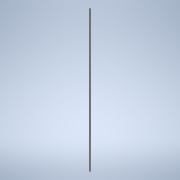
# Autodesk Inventor part: ball screw
Saved by Autodesk Inventor 2020 (Build 240168000, 168)
## iProperties
Created: 2020-07-28
Part Number: ball screw
Material: Stainless Steel
Document SubType Name: Modeling
Designer: Vikki
Density: 8 g/cm^3
Appearance: Semi-Polished
Mass: 1603.28 g
Surface Area: 506.216 cm^2
Volume: 200.409 cm^3
Author: Vikki
Autodesk Inventor part; units mm, degrees
ref_plane "YZ Plane" through (0, 0, 0) normal (1, 0, 0) x (0, 1, 0)
ref_plane "XZ Plane" through (0, 0, 0) normal (0, 1, 0) x (-1, 0, 0)
ref_plane "XY Plane" through (0, 0, 0) normal (0, 0, 1) x (1, 0, 0)
sketch "Sketch1" plane through (0, 0, 0) normal (0, 1, 0) x (-1, 0, 0)
  circle A0 centre (0, 0) radius 5
  dimension "d0" = 10
  constraints: 1 centre point, 1 coincident
  measures "d0" diameter of A0
extrude "Extrusion1" add sketch "Sketch1" along normal blind 1000
sketch "Sketch2" plane through (0, 1000, 0) normal (0, 1, 0) x (1, 0, 0)
  circle A0 centre (0, 0) radius 5 projected
  circle A1 centre (0, 0) radius 5 projected
  line L0 (5, 0) -> (5, 0)
  line L1 (0, 0) -> (0, 5)
  point P0 (5, 6.245)
  point P1 (5, -6.245)
  dimension "d3" = 5
  constraints: 4 end point, 2 point on circle, 1 parallel, 1 vertical
  measures "d3" distance from line of L0 point (0, 0)
extrude "Extrusion2" [suppressed]
thread "Thread1" size "M60x4" class "6g" standard "ANSI Metric M Profile" length 975
body "Solid1"
